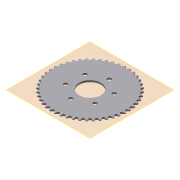
# Autodesk Inventor part: 25 sprocket 48T
Saved by Autodesk Inventor 2011 (Build 150239000, 239)
## iProperties
Created: 2011-07-15
Part Number: 25 sprocket 48T
Material: Aluminum-6061
Document SubType Name: Modeling
Designer: Dan Niemitalo
Density: 2.71 g/cm^3
Mass: 40.3507 g
Surface Area: 144.824 cm^2
Volume: 14.8896 cm^3
CustomPartVersion: 1
Author: Dan Niemitalo
Autodesk Inventor part; units mm, degrees
ref_plane "YZ Plane" through (0, 0, 0) normal (1, 0, 0) x (0, 1, 0)
ref_plane "XZ Plane" through (0, 0, 0) normal (0, 1, 0) x (-1, 0, 0)
sketch "Theoretical Tooth Profile" plane through (0, 0, 0) normal (0, 0, 1) x (1, 0, 0)
  circle A0 centre (0, 0) radius 48.5451 construction
  line L0 (0, 0) -> (0, 48.5451) construction
  line L1 (0, 0) -> (6.3364, 48.1298) construction
  circle A1 centre (0, 0) radius 50.3461
  arc A2 (-1.3688, 47.5414) -> (1.3688, 47.5414) centre (0, 48.5451) ccw
  line L2 (0, 48.5451) -> (6.3364, 48.1298) construction
  line L3 (0, 48.5451) -> (2.1303, 50.1071) construction
  line L4 (2.1303, 50.1071) -> (-1.9619, 48.6647) construction
  arc A3 (2.9113, 50.2619) -> (2.1226, 49.1205) centre (4.6129, 48.2427) ccw
  arc A4 (-2.1226, 49.1205) -> (-2.9113, 50.2619) centre (-4.6129, 48.2427) ccw
  line L5 (-4.6129, 48.2427) -> (-2.1226, 49.1205) construction
  arc A5 (-1.9619, 48.6647) -> (-1.3688, 47.5414) centre (2.1303, 50.1071) ccw
  line L6 (-1.9619, 48.6647) -> (-2.1226, 49.1205)
  arc A6 (1.3688, 47.5414) -> (1.9619, 48.6647) centre (-2.1303, 50.1071) ccw
  line L7 (2.1226, 49.1205) -> (1.9619, 48.6647)
  line L8 (0, 0) -> (3.2928, 50.2383) construction
  point P0 (3.1682, 48.3374)
  dimension "d0" = 97.0902
  dimension "d2" = 7.5
  dimension "d3" = 1.6973
  dimension "d10" = 126.25
  dimension "d11" = 16.833
  dimension "d12" = 2.6416
  dimension "d13" = 4.339
  dimension "d14" = 4.6228
  dimension "d23" = 1.905
  constraints: 18 end point, 15 point on circle, 7 centre point, 3 coincident, 3 point on line, 3 symmetric about line, 3 tangent, 1 equal radius, 1 midpoint, 1 parallel, 1 vertical, 1 other
  measures "d0" diameter of A0
  measures "d2" angle of L1 L0
  measures "d3" radius of A2
  measures "d10" angle of L3 L0
  measures "d11" angle of L4 L3
  measures "d12" distance of L2.start L3.end
  measures "d13" distance of L3.end L4.end
  measures "d14" distance of A3.centre L0.end
  measures "d23" distance from line of L8.end L2
sketch "Tooth Profile" plane through (0, 0, 0) normal (0, 0, 1) x (1, 0, 0)
  circle A0 centre (0, 0) radius 50.3461 projected
  line L0 (0, 0) -> (0, 48.5451) construction
  line L1 (0, 48.5451) -> (1.5853, 47.9385) construction
  arc A1 (-1.5853, 47.9385) -> (1.5853, 47.9385) centre (0, 48.5451) ccw
  line L2 (-1.5853, 47.9385) -> (0, 48.5451) construction
  arc A2 (-1.5853, 47.9385) -> (-2.6583, 50.2759) centre (-20.0891, 40.8587) ccw
  arc A3 (2.6583, 50.2759) -> (1.5853, 47.9385) centre (20.0891, 40.8587) ccw
  dimension "d44" = 138.125
  dimension "d45" = 1.6973
  dimension "d46" = 19.812
  constraints: 8 point on circle, 7 end point, 3 centre point, 2 tangent, 1 coincident, 1 equal radius, 1 symmetric about line, 1 vertical
  measures "d44" angle of L1 L2
  measures "d45" radius of A1
  measures "d46" radius of A3
sketch "Section Profile" plane through (0, 0, 0) normal (1, 0, 0) x (0, 1, 0)
  line L0 (50.3461, 0) -> (-50.3461, 0) projected
  line L1 (44.6311, 1.143) -> (-44.6311, 1.143)
  line L2 (-44.6311, 1.143) -> (-44.6311, -1.143)
  line L3 (-44.6311, -1.143) -> (44.6311, -1.143)
  line L4 (44.6311, -1.143) -> (44.6311, 1.143)
  line L5 (44.6311, 1.143) -> (50.3461, 1.143) construction
  line L6 (50.3461, 1.143) -> (50.3461, -1.143) construction
  line L7 (50.3461, -1.143) -> (44.6311, -1.143) construction
  line L8 (44.6311, -1.143) -> (44.6311, 1.143)
  arc A0 (50.3461, 0.3492) -> (47.1703, 1.143) centre (47.1703, -5.6071) ccw
  arc A1 (47.1703, -1.143) -> (50.3461, -0.3492) centre (47.1703, 5.6071) ccw
  line L9 (47.1703, 1.143) -> (0, 1.143)
  line L10 (0, 1.143) -> (0, -1.143)
  line L11 (0, -1.143) -> (47.1703, -1.143)
  line L12 (0, 1.143) -> (0, -1.143)
  line L13 (50.3461, 0.3492) -> (50.3461, -0.3492)
  point P0 (0, 0)
  point P1 (0, 0)
  dimension "d30" = 2.286
  dimension "d31" = 89.2623
  dimension "d32" = 2.286
  dimension "d33" = 0.7937
  dimension "d34" = 6.75
  dimension "d43" = 1.143
  constraints: 26 end point, 7 midpoint, 5 perpendicular, 4 parallel, 4 point on circle, 3 point on line, 3 symmetric about line, 2 centre point, 2 horizontal, 2 tangent, 1 collinear, 1 other
  measures "d30" distance between parallel lines of L7 L5
  measures "d31" distance between parallel lines of L2 L4
  measures "d32" distance between parallel lines of L3 L1
  measures "d33" distance from line of L13.start L5
  measures "d34" radius of A0
  measures "d43" distance between parallel lines of L3 L0
revolve "Shroud" add sketch "Section Profile" angle 360 about axis through (0, 0, 1.143) along (0, 0, -1) contours L10 L3 L2 L0 | L0 L2 L1 L10
revolve "Strand" add sketch "Section Profile" angle 360 about axis through (0, 0, 1.143) along (0, 0, -1) contours L13 A1 L11 L4 L0 | L0 L4 L9 A0 L13 | L4 L3 L10 L0 | L0 L10 L1 L4
pattern_of_one "Strand Pattern"
extrude "Theoretical Tooth" cut sketch "Theoretical Tooth Profile" along normal through all both and the other way through all contours A3 L7 A6 A2 A5 L6 A4 A1 picked at (-0.3236, 48.7095)
extrude "Tooth" [suppressed]
pattern_circular "Tooth Pattern" count 48 over 360 about axis through (0, 0, -10) along (0, 0, 1) of "Theoretical Tooth"
ref_plane "Timing Plane" through (0, 48.5451, 0) normal (1, 0, 0) x (0, 1, 0)
sketch "Sketch4" plane through (0, 0, 1.143) normal (0, 0, 1) x (0.9978589, -0.0654031, 0)
  arc A0 (2.1052, 47.1233) -> (-2.1052, 47.1233) centre (0, 0) ccw projected
  arc A1 (8.238, 46.4454) -> (4.0636, 46.995) centre (0, 0) ccw projected
  circle A2 centre (0, 0) radius 14.2812
  dimension "d51" = 28.5623
  constraints: 1 centre point, 1 coincident
  measures "d51" diameter of A2
hole "Hole1" at (0, 0, 1.143) direction (0, 0, -1) diameter 28.5623 end through all
sketch "Sketch5" plane through (0, 0, 1.143) normal (0, 0, 1) x (0.9978589, -0.0654031, 0)
  arc A0 (8.238, 46.4454) -> (4.0636, 46.995) centre (0, 0) ccw projected
  circle A1 centre (0, 0) radius 23.8125 construction
  circle A2 centre (-0.0023, 23.8125) radius 2.6162
  circle A3 centre (-20.6234, 11.9043) radius 2.6162
  circle A4 centre (-20.6211, -11.9082) radius 2.6162
  circle A5 centre (0.0023, -23.8125) radius 2.6162
  circle A6 centre (20.6234, -11.9043) radius 2.6162
  circle A7 centre (20.6211, 11.9082) radius 2.6162
  dimension "d59" = 47.625
  dimension "d60" = 5.2324
  dimension "d63" = 360
  constraints: 6 centre point, 1 coincident, 16 other
  measures "d60" diameter of A2
hole "Hole2" at (1.5551, 23.7617, 1.143) at (21.3558, 10.5341, 1.143) at (19.8006, -13.2276, 1.143) at (-1.5551, -23.7617, 1.143) at (-21.3558, -10.5341, 1.143) at (-19.8006, 13.2276, 1.143) direction (0, 0, -1) diameter 5.2324 end through all
equation "\"d3\" = 0.5 * da_Dr + da_SC"
equation "\"d12\" = 0.8 * da_Dr"
equation "\"d13\" = 1.3 * da_Dr + da_SC"
equation "\"d14\" = 1.4 * da_Dr"
equation "\"d23\" = da_Ha"
equation "\"d44\" = da_Alfa"
equation "\"d45\" = da_Ri"
equation "\"d46\" = da_Re"
equation "\"d30\" = da_Bf"
equation "\"d31\" = da_Ds"
equation "\"d32\" = da_Bs"
equation "\"d33\" = da_Ba"
equation "\"d34\" = da_Rx"
equation "\"d40\" = da_pt"
equation "\"form_type\" = 0"
equation "\"da_p\" = 6.35"
equation "\"da_Dr\" = 3.302"
equation "\"da_SC\" = 0.04636"
equation "\"da_Ha\" = 1.905"
equation "\"da_pt\" = 6.4008"
equation "\"da_Bf\" = 2.286"
equation "\"da_Ba\" = 0.79375"
equation "\"da_Rx\" = 6.75005"
equation "\"da_Ra\" = 0.254"
equation "\"da_Bs\" = 2.286"
equation "\"da_Ds\" = 89.26228"
equation "\"da_Re\" = 19.812"
equation "\"da_Ri\" = 1.69735"
equation "\"da_Alfa\" = 138.125deg"
body "Solid1"
